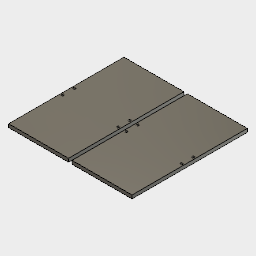
jalkalevyt transformer v1 (Autodesk Fusion 360 design; units mm, degrees)
Autodesk Fusion 360 part; units mm, degrees
box "BoxPrimitive5" add length 100 width 52 height 3 placed x (0, 0, -1) y (-1, 0, 0) z (0, 1, 0) at (62, 0, 85) makes body 1
hole "Hole6" at (12, 3, 40) direction (0, -1, 0) diameter 2 depth 20 tip angle 118 bodies 1
hole "Hole7" at (12, 3, 30) direction (0, -1, 0) diameter 2 depth 20 tip angle 118 bodies 1
hole "Hole8" at (60, 3, 40) direction (0, -1, 0) diameter 2 depth 20 tip angle 118 bodies 1
hole "Hole9" at (60, 3, 30) direction (0, -1, 0) diameter 2 depth 20 tip angle 118 bodies 1
copy_body "CopyPasteBodies3" bodies 1 makes body 2
move_body "Move20" bodies 2 to x (1, 0, 0) y (0, 1, 0) z (0, 0, 1) at (-65, 0, 0)
move_body "Move21" bodies 1 to x (1, 0, 0) y (0, 1, 0) z (0, 0, 1) at (-10, 0, 0)
